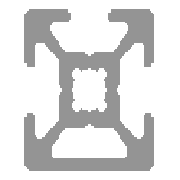
# Autodesk Inventor part: 3 842 992 889-2mm
Saved by Autodesk Inventor 2011 SP1 (Build 150282100, 282)
## iProperties
Created: 2011-02-10
Part Number: 3 842 992 889-2mm
Document SubType Name: Modeling
Designer: S. Wile
Density: 2.71 g/cm^3
Categories: <MemberInstance><Categories><Category DisplayName="Structural Shapes" InternalName="089c4875-fa83-4c05-b084-43b9cc11f5ed" Mnemonic="GRDR"><CategoryParameter DisplayName="Custom Base Point" InternalName="4f1d1b73-316d-484b-a3df-9cbabb16eb77" Mnemonic="shpBasePoint"/><CategoryParameter DisplayName="FG Authored" InternalName="9c666724-f362-4ea7-ac62-f6a007de5c69" Mnemonic="shpFGAuto"/><CategoryParameter DisplayName="Legacy Member ID" InternalName="340afe4f-75d7-48d3-ab7d-943f3c3da468" Mnemonic="LegacyMemberID"/><CategoryParameter DisplayName="Base Length" InternalName="42e34263-8f20-4d0e-ad48-bf1385b87c24" Mnemonic="shplen"/><CategoryParameter DisplayName="Distance of the Center of Gravity X-X" InternalName="26c9bdb8-9c79-4b4f-a92e-8e197583c9c4" Mnemonic="grcendistX"/><CategoryParameter DisplayName="Distance of the Center of Gravity Y-Y" InternalName="bcc4fb17-7af4-436a-8f8c-d0aa3b0248c5" Mnemonic="grcendistY"/><CategoryParameter DisplayName="Torsional Rigidity Modulus" InternalName="26c1ec35-5026-4c63-ad0a-751cf684a536" Mnemonic="torrigmod"/><CategoryParameter DisplayName="Torsional Section Modulus" InternalName="7c55a8dc-8844-49f9-a867-cc677b30ec9a" Mnemonic="torsecmod"/><CategoryParameter DisplayName="Coefficient of Shear Displacement" InternalName="de4c90c6-aaa8-468f-a335-6737b311b5d3" Mnemonic="shdispc"/><CategoryParameter DisplayName="Section Area" InternalName="1ff91680-64b0-4202-b9a3-7fd3f94bba3b" Mnemonic="secarea"/><CategoryParameter DisplayName="Moment of Inertia (x)" InternalName="4cd780bc-73d7-43ac-917a-579e5cbd684d" Mnemonic="inermomx"/><CategoryParameter DisplayName="Moment of Inertia (y)" InternalName="4b9f58ea-bced-460e-81ea-3d29ca5a49e3" Mnemonic="inermomy"/><CategoryParameter DisplayName="Section Module (x)" InternalName="72cfad18-cf51-4ed4-aaa7-c6b224f8419f" Mnemonic="secmodx"/><CategoryParameter DisplayName="Section Module (y)" InternalName="59eaa5e9-d227-48dc-b6c1-6920f96e0f95" Mnemonic="secmody"/><CategoryParameter DisplayName="Radius of Gyration (x)" InternalName="25778675-03e9-40c1-b6a8-4a9ed693320d" Mnemonic="gyrradx"/><CategoryParameter DisplayName="Radius of Gyration (y)" InternalName="bfa18ebe-1636-4dbe-8d42-b263e0b73184" Mnemonic="gyrrady"/><CategoryParameter DisplayName="Shape Thickness" InternalName="d109cf76-8eb4-42fc-9800-4409734adc67" Mnemonic="shpthick"/><CategoryParameter DisplayName="Second Shape Thickness" InternalName="9251a8e1-85fd-4e47-af99-afdb762317d9" Mnemonic="shpthick2"/><CategoryParameter DisplayName="Shape Width" InternalName="7c717d54-a18f-4666-b4d4-573cce22c62c" Mnemonic="shpwdth"/><CategoryParameter DisplayName="Shape Height" InternalName="50274e7d-5ac0-4796-92cb-c59e54983c67" Mnemonic="shpheig"/><CategoryParameter DisplayName="Mass per Length Unit" InternalName="0bb95a10-148f-4027-a459-38d7b056702a" Mnemonic="shpmass"/><CategoryParameter DisplayName="Section Designation" InternalName="5a64d034-428d-49c8-ba32-7619764de20f" Mnemonic="shpdes"/><Category DisplayName="Other" InternalName="f02205ff-2390-476f-921c-0b3185f88e84" Mnemonic="OTHSHP"><CategoryParameter DisplayName="Moment of Inertia (x)" InternalName="ec6737bc-264f-43ed-b0bd-f6d410c2718d" Mnemonic="inermomx"/><CategoryParameter DisplayName="Moment of Inertia (y)" InternalName="044c654e-f649-48ac-84cc-650a29ae31ca" Mnemonic="inermomy"/><CategoryParameter DisplayName="Section Module (x)" InternalName="cac70804-9d39-43bb-be17-56ea1f39a6c2" Mnemonic="secmodx"/><CategoryParameter DisplayName="Section Module (y)" InternalName="88b8bff9-a616-4028-93d5-ed4f79680d13" Mnemonic="secmody"/><CategoryParameter DisplayName="Section Area" InternalName="c46ecdf8-b6eb-4db9-8b25-30258930c1e3" Mnemonic="secarea"/><CategoryParameter DisplayName="Radius of Gyration (x)" InternalName="ee72c61e-565e-4fd6-b448-66e1e1abcb7e" Mnemonic="gyrradx"/><CategoryParameter DisplayName="Radius of Gyration (y)" InternalName="743e1dfe-1bba-408b-b985-cf752b207386" Mnemonic="gyrrady"/><CategoryParameter DisplayName="Shape Thickness" InternalName="12b1a788-9233-48fd-a933-2df8ff42b15f" Mnemonic="shpthick"/><CategoryParameter DisplayName="Mass per Length Unit" InternalName="2fd289d6-9394-4d2d-97e6-6659d7d4551d" Mnemonic="shpmass"/></Category></Category></Categories><FamilyTemplate Id="20x20-3S"><FamilyTemplateParameters><FamilyTemplateParameter ObjectType="kUserParameterObject" ValueType="xs:double" Id="1" ObjectReferenceKey="G_L"/><FamilyTemplateParameter ObjectType="kUserParameterObject" ValueType="xs:double" Id="2" ObjectReferenceKey="G_OFFSET_END"/><FamilyTemplateParameter ObjectType="kUserParameterObject" ValueType="xs:double" Id="3" ObjectReferenceKey="G_OFFSET_START"/><FamilyTemplateParameter ObjectType="kUserParameterObject" ValueType="xs:double" Id="4" ObjectReferenceKey="Length"/><FamilyTemplateParameter ObjectType="kPropertyObject" ValueType="xs:string" Id="7" ObjectReferenceKey="{32853F0F-3444-11d1-9E93-0060B03C1CA6}" SubObjectId="52"/><FamilyTemplateParameter ObjectType="kPartComponentDefinitionObject" ValueType="xs:string" Id="8" SubObjectId="Material"/><FamilyTemplateParameter ObjectType="kPropertyObject" ValueType="xs:string" Id="9" ObjectReferenceKey="{32853F0F-3444-11d1-9E93-0060B03C1CA6}" SubObjectId="5"/><FamilyTemplateParameter ObjectType="kPropertyObject" ValueType="xs:string" Id="10" ObjectReferenceKey="{32853F0F-3444-11D1-9E93-0060B03C1CA6}" SubObjectId="55"/><FamilyTemplateParameter ObjectType="kiPartTableColumnObject" ValueType="xs:string" Id="21" ObjectReferenceKey="FILENAME"/><FamilyTemplateParameter ObjectType="kiPartTableColumnObject" ValueType="xs:string" Id="22" ObjectReferenceKey="MEMBER_REVISION"/></FamilyTemplateParameters></FamilyTemplate><CategoryParameterMap><ParamToTemplateMap><ParamToTemplate CategoryParameter="//CategoryParameter[@InternalName='9c666724-f362-4ea7-ac62-f6a007de5c69']" ConstantValue="1"/><ParamToTemplate CategoryParameter="//CategoryParameter[@InternalName='2675968c-4ce5-49e0-a4f5-552d29089031']" TemplateParameter="7"/><ParamToTemplate CategoryParameter="//CategoryParameter[@InternalName='8b46a4cc-9585-4fed-90c3-899f57e09a73']" TemplateParameter="21"/><ParamToTemplate CategoryParameter="//CategoryParameter[@InternalName='42e34263-8f20-4d0e-ad48-bf1385b87c24']" TemplateParameter="4"/><ParamToTemplate CategoryParameter="//CategoryParameter[@InternalName='818a152a-d3c3-49ca-80ee-df7d91421b8e']" TemplateParameter="8"/><ParamToTemplate CategoryParameter="//CategoryParameter[@InternalName='a65d44b9-392f-4f4f-857b-e4b3d54996fe']" TemplateParameter="22"/><ParamToTemplate CategoryParameter="//CategoryParameter[@InternalName='016b6077-bfbe-49bd-92c9-d8d59c39c941']" TemplateParameter="9"/></ParamToTemplateMap></CategoryParameterMap></MemberInstance>
Stock Number: 3 842 992 889
Description: PROFILE 20x20 3S, -/-
Material: Aluminum-6061
Mass: 0.942693 g
Surface Area: 7.19171 cm^2
Volume: 0.347857 cm^3
Author: S. Wile
Autodesk Inventor part; units mm, degrees
ref_plane "YZ Plane" through (0, 0, 0) normal (1, 0, 0) x (0, 1, 0)
ref_plane "XZ Plane" through (0, 0, 0) normal (0, 1, 0) x (-1, 0, 0)
ref_plane "XY Plane" through (0, 0, 0) normal (0, 0, 1) x (1, 0, 0)
sketch "20x20-3S" plane through (0, 0, 0) normal (0, 0, 1) x (1, 0, 0)
  arc A0 (45.4955, 77.845) -> (45.5955, 77.8718) centre (45.4955, 78.045) ccw
  line L0 (45.4955, 77.845) -> (43.2168, 77.845)
  arc A1 (43.2168, 77.845) -> (42.8633, 77.6986) centre (43.2168, 77.345) ccw
  line L1 (42.8633, 77.6986) -> (40.5955, 75.4308)
  arc A2 (40.5955, 75.4308) -> (40.4491, 75.0772) centre (40.9491, 75.0772) ccw
  line L2 (40.4491, 75.0772) -> (40.4491, 74.345)
  arc A3 (40.4491, 74.345) -> (40.9491, 73.845) centre (40.9491, 74.345) ccw
  line L3 (40.9491, 73.845) -> (51.9491, 73.845)
  arc A4 (51.9491, 73.845) -> (52.4491, 74.345) centre (51.9491, 74.345) ccw
  line L4 (52.4491, 74.345) -> (52.4491, 75.0772)
  line L5 (55.4491, 85.295) -> (55.7491, 85.295)
  arc A5 (54.9491, 85.795) -> (55.4491, 85.295) centre (55.4491, 85.795) ccw
  line L6 (54.9491, 87.845) -> (54.9491, 85.795)
  arc A6 (54.9491, 87.845) -> (54.4491, 88.345) centre (54.4491, 87.845) ccw
  line L7 (53.7168, 88.345) -> (54.4491, 88.345)
  arc A7 (53.7168, 88.345) -> (53.3633, 88.1986) centre (53.7168, 87.845) ccw
  line L8 (51.0955, 85.9308) -> (53.3633, 88.1986)
  arc A8 (51.0955, 85.9308) -> (50.9491, 85.5772) centre (51.4491, 85.5772) ccw
  line L9 (50.9491, 83.2986) -> (50.9491, 85.5772)
  arc A9 (50.9223, 83.1986) -> (50.9491, 83.2986) centre (50.7491, 83.2986) ccw
  line L10 (50.4872, 82.445) -> (50.9223, 83.1986)
  arc A10 (50.4872, 82.445) -> (50.4872, 82.245) centre (50.6604, 82.345) ccw
  line L11 (50.9223, 81.4914) -> (50.4872, 82.245)
  arc A11 (50.9491, 81.3914) -> (50.9223, 81.4914) centre (50.7491, 81.3914) ccw
  line L12 (50.9491, 79.1128) -> (50.9491, 81.3914)
  arc A12 (50.9491, 79.1128) -> (51.0955, 78.7592) centre (51.4491, 79.1128) ccw
  line L13 (53.3633, 76.4915) -> (51.0955, 78.7592)
  arc A13 (53.3633, 76.4915) -> (53.7168, 76.345) centre (53.7168, 76.845) ccw
  line L14 (54.4491, 76.345) -> (53.7168, 76.345)
  arc A14 (54.4491, 76.345) -> (54.9491, 76.845) centre (54.4491, 76.845) ccw
  line L15 (54.9491, 78.795) -> (54.9491, 76.845)
  arc A15 (55.4491, 79.295) -> (54.9491, 78.795) centre (55.4491, 78.795) ccw
  line L16 (55.7491, 79.295) -> (55.4491, 79.295)
  arc A16 (55.9491, 79.095) -> (55.7491, 79.295) centre (55.7491, 79.095) ccw
  line L17 (55.9491, 78.995) -> (55.9491, 79.095)
  arc A17 (55.9491, 78.995) -> (56.1491, 78.795) centre (56.1491, 78.995) ccw
  line L18 (56.2491, 78.795) -> (56.1491, 78.795)
  arc A18 (56.4491, 78.595) -> (56.2491, 78.795) centre (56.2491, 78.595) ccw
  line L19 (56.4491, 73.845) -> (56.4491, 78.595)
  arc A19 (54.9491, 72.345) -> (56.4491, 73.845) centre (54.9491, 73.845) ccw
  line L20 (37.9491, 72.345) -> (54.9491, 72.345)
  arc A20 (36.4491, 73.845) -> (37.9491, 72.345) centre (37.9491, 73.845) ccw
  line L21 (36.4491, 78.595) -> (36.4491, 73.845)
  arc A21 (36.6491, 78.795) -> (36.4491, 78.595) centre (36.6491, 78.595) ccw
  line L22 (36.7491, 78.795) -> (36.6491, 78.795)
  arc A22 (36.7491, 78.795) -> (36.9491, 78.995) centre (36.7491, 78.995) ccw
  line L23 (36.9491, 79.095) -> (36.9491, 78.995)
  arc A23 (37.1491, 79.295) -> (36.9491, 79.095) centre (37.1491, 79.095) ccw
  line L24 (37.4491, 79.295) -> (37.1491, 79.295)
  arc A24 (37.9491, 78.795) -> (37.4491, 79.295) centre (37.4491, 78.795) ccw
  line L25 (37.9491, 76.845) -> (37.9491, 78.795)
  arc A25 (37.9491, 76.845) -> (38.4491, 76.345) centre (38.4491, 76.845) ccw
  line L26 (39.1813, 76.345) -> (38.4491, 76.345)
  arc A26 (39.1813, 76.345) -> (39.5349, 76.4915) centre (39.1813, 76.845) ccw
  line L27 (41.8026, 78.7592) -> (39.5349, 76.4915)
  arc A27 (41.8026, 78.7592) -> (41.9491, 79.1128) centre (41.4491, 79.1128) ccw
  line L28 (41.9491, 81.3914) -> (41.9491, 79.1128)
  arc A28 (41.9759, 81.4914) -> (41.9491, 81.3914) centre (42.1491, 81.3914) ccw
  line L29 (42.4109, 82.245) -> (41.9759, 81.4914)
  arc A29 (42.4109, 82.245) -> (42.4109, 82.445) centre (42.2377, 82.345) ccw
  line L30 (41.9759, 83.1986) -> (42.4109, 82.445)
  arc A30 (41.9491, 83.2986) -> (41.9759, 83.1986) centre (42.1491, 83.2986) ccw
  line L31 (41.9491, 85.5772) -> (41.9491, 83.2986)
  arc A31 (41.9491, 85.5772) -> (41.8026, 85.9308) centre (41.4491, 85.5772) ccw
  line L32 (39.5349, 88.1986) -> (41.8026, 85.9308)
  arc A32 (39.5349, 88.1986) -> (39.1813, 88.345) centre (39.1813, 87.845) ccw
  line L33 (38.4491, 88.345) -> (39.1813, 88.345)
  arc A33 (38.4491, 88.345) -> (37.9491, 87.845) centre (38.4491, 87.845) ccw
  line L34 (37.9491, 85.795) -> (37.9491, 87.845)
  arc A34 (37.4491, 85.295) -> (37.9491, 85.795) centre (37.4491, 85.795) ccw
  line L35 (37.1491, 85.295) -> (37.4491, 85.295)
  arc A35 (36.9491, 85.495) -> (37.1491, 85.295) centre (37.1491, 85.495) ccw
  line L36 (36.9491, 85.695) -> (36.9491, 85.495)
  arc A36 (36.9491, 85.695) -> (36.7491, 85.895) centre (36.7491, 85.695) ccw
  line L37 (36.6491, 85.895) -> (36.7491, 85.895)
  arc A37 (36.4491, 86.095) -> (36.6491, 85.895) centre (36.6491, 86.095) ccw
  line L38 (36.4491, 90.845) -> (36.4491, 86.095)
  arc A38 (37.9491, 92.345) -> (36.4491, 90.845) centre (37.9491, 90.845) ccw
  line L39 (42.6991, 92.345) -> (37.9491, 92.345)
  arc A39 (42.8991, 92.145) -> (42.6991, 92.345) centre (42.6991, 92.145) ccw
  line L40 (42.8991, 92.045) -> (42.8991, 92.145)
  arc A40 (42.8991, 92.045) -> (43.0991, 91.845) centre (43.0991, 92.045) ccw
  line L41 (43.2491, 91.845) -> (43.0991, 91.845)
  arc A41 (43.4491, 91.645) -> (43.2491, 91.845) centre (43.2491, 91.645) ccw
  line L42 (43.4491, 91.345) -> (43.4491, 91.645)
  arc A42 (42.9491, 90.845) -> (43.4491, 91.345) centre (42.9491, 91.345) ccw
  line L43 (40.9491, 90.845) -> (42.9491, 90.845)
  arc A43 (40.9491, 90.845) -> (40.4491, 90.345) centre (40.9491, 90.345) ccw
  line L44 (40.4491, 89.6128) -> (40.4491, 90.345)
  arc A44 (40.4491, 89.6128) -> (40.5955, 89.2592) centre (40.9491, 89.6128) ccw
  line L45 (42.8633, 86.9915) -> (40.5955, 89.2592)
  arc A45 (42.8633, 86.9915) -> (43.2168, 86.845) centre (43.2168, 87.345) ccw
  line L46 (45.4955, 86.845) -> (43.2168, 86.845)
  arc A46 (45.5955, 86.8182) -> (45.4955, 86.845) centre (45.4955, 86.645) ccw
  line L47 (46.3491, 86.3831) -> (45.5955, 86.8182)
  arc A47 (46.3491, 86.3831) -> (46.5491, 86.3831) centre (46.4491, 86.5563) ccw
  arc A48 (52.4491, 75.0772) -> (52.3026, 75.4308) centre (51.9491, 75.0772) ccw
  line L48 (52.3026, 75.4308) -> (50.0349, 77.6986)
  arc A49 (50.0349, 77.6986) -> (49.6813, 77.845) centre (49.6813, 77.345) ccw
  line L49 (49.6813, 77.845) -> (47.4027, 77.845)
  arc A50 (47.3027, 77.8718) -> (47.4027, 77.845) centre (47.4027, 78.045) ccw
  line L50 (47.3027, 77.8718) -> (46.5491, 78.3069)
  arc A51 (46.5491, 78.3069) -> (46.3491, 78.3069) centre (46.4491, 78.1337) ccw
  line L51 (46.3491, 78.3069) -> (45.5955, 77.8718)
  arc A52 (44.562, 85.2927) -> (43.5014, 84.2321) centre (46.4491, 82.345) ccw
  line L52 (43.5014, 84.2321) -> (44.0482, 83.5803)
  arc A53 (44.0482, 83.5803) -> (44.0482, 81.1097) centre (46.4491, 82.345) ccw
  line L53 (44.0482, 81.1097) -> (43.5014, 80.458)
  arc A54 (43.5014, 80.458) -> (44.562, 79.3973) centre (46.4491, 82.345) ccw
  line L54 (44.562, 79.3973) -> (45.2138, 79.9442)
  arc A55 (45.2138, 79.9442) -> (47.6844, 79.9442) centre (46.4491, 82.345) ccw
  line L55 (47.6844, 79.9442) -> (48.3361, 79.3973)
  arc A56 (48.3361, 79.3973) -> (49.3968, 80.458) centre (46.4491, 82.345) ccw
  line L56 (49.3968, 80.458) -> (48.8499, 81.1097)
  arc A57 (48.8499, 81.1097) -> (48.8499, 83.5803) centre (46.4491, 82.345) ccw
  line L57 (48.8499, 83.5803) -> (49.3968, 84.2321)
  arc A58 (49.3968, 84.2321) -> (48.3361, 85.2927) centre (46.4491, 82.345) ccw
  line L58 (48.3361, 85.2927) -> (47.6844, 84.7458)
  arc A59 (47.6844, 84.7458) -> (45.2138, 84.7458) centre (46.4491, 82.345) ccw
  line L59 (45.2138, 84.7458) -> (44.562, 85.2927)
  line L60 (47.3027, 86.8182) -> (46.5491, 86.3831)
  arc A60 (47.4027, 86.845) -> (47.3027, 86.8182) centre (47.4027, 86.645) ccw
  line L61 (49.6813, 86.845) -> (47.4027, 86.845)
  arc A61 (49.6813, 86.845) -> (50.0349, 86.9915) centre (49.6813, 87.345) ccw
  line L62 (52.3026, 89.2592) -> (50.0349, 86.9915)
  arc A62 (52.3026, 89.2592) -> (52.4491, 89.6128) centre (51.9491, 89.6128) ccw
  line L63 (52.4491, 90.345) -> (52.4491, 89.6128)
  arc A63 (52.4491, 90.345) -> (51.9491, 90.845) centre (51.9491, 90.345) ccw
  line L64 (49.9491, 90.845) -> (51.9491, 90.845)
  arc A64 (49.4491, 91.345) -> (49.9491, 90.845) centre (49.9491, 91.345) ccw
  line L65 (49.4491, 91.645) -> (49.4491, 91.345)
  arc A65 (49.6491, 91.845) -> (49.4491, 91.645) centre (49.6491, 91.645) ccw
  line L66 (49.7991, 91.845) -> (49.6491, 91.845)
  arc A66 (49.7991, 91.845) -> (49.9991, 92.045) centre (49.7991, 92.045) ccw
  line L67 (49.9991, 92.145) -> (49.9991, 92.045)
  arc A67 (50.1991, 92.345) -> (49.9991, 92.145) centre (50.1991, 92.145) ccw
  line L68 (54.9491, 92.345) -> (50.1991, 92.345)
  arc A68 (56.4491, 90.845) -> (54.9491, 92.345) centre (54.9491, 90.845) ccw
  line L69 (56.4491, 86.095) -> (56.4491, 90.845)
  arc A69 (56.2491, 85.895) -> (56.4491, 86.095) centre (56.2491, 86.095) ccw
  line L70 (56.1491, 85.895) -> (56.2491, 85.895)
  arc A70 (56.1491, 85.895) -> (55.9491, 85.695) centre (56.1491, 85.695) ccw
  line L71 (55.9491, 85.495) -> (55.9491, 85.695)
  arc A71 (55.7491, 85.295) -> (55.9491, 85.495) centre (55.7491, 85.495) ccw
sketch "Sketch1" plane through (0, 0, 0) normal (0, 0, 1) x (1, 0, 0)
  arc A0 (-0.9536, -4.5) -> (-0.8536, -4.4732) centre (-0.9536, -4.3) ccw
  line L0 (-0.9536, -4.5) -> (-3.2322, -4.5)
  arc A1 (-3.2322, -4.5) -> (-3.5858, -4.6464) centre (-3.2322, -5) ccw
  line L1 (-3.5858, -4.6464) -> (-5.8536, -6.9142)
  arc A2 (-5.8536, -6.9142) -> (-6, -7.2678) centre (-5.5, -7.2678) ccw
  line L2 (-6, -7.2678) -> (-6, -8)
  arc A3 (-6, -8) -> (-5.5, -8.5) centre (-5.5, -8) ccw
  line L3 (-5.5, -8.5) -> (5.5, -8.5)
  arc A4 (5.5, -8.5) -> (6, -8) centre (5.5, -8) ccw
  line L4 (6, -8) -> (6, -7.2678)
  line L5 (9, 2.95) -> (9.3, 2.95)
  arc A5 (8.5, 3.45) -> (9, 2.95) centre (9, 3.45) ccw
  line L6 (8.5, 5.5) -> (8.5, 3.45)
  arc A6 (8.5, 5.5) -> (8, 6) centre (8, 5.5) ccw
  line L7 (7.2678, 6) -> (8, 6)
  arc A7 (7.2678, 6) -> (6.9142, 5.8536) centre (7.2678, 5.5) ccw
  line L8 (4.6464, 3.5858) -> (6.9142, 5.8536)
  arc A8 (4.6464, 3.5858) -> (4.5, 3.2322) centre (5, 3.2322) ccw
  line L9 (4.5, 0.9536) -> (4.5, 3.2322)
  arc A9 (4.4732, 0.8536) -> (4.5, 0.9536) centre (4.3, 0.9536) ccw
  line L10 (4.0381, 0.1) -> (4.4732, 0.8536)
  arc A10 (4.0381, 0.1) -> (4.0381, -0.1) centre (4.2113, 0) ccw
  line L11 (4.4732, -0.8536) -> (4.0381, -0.1)
  arc A11 (4.5, -0.9536) -> (4.4732, -0.8536) centre (4.3, -0.9536) ccw
  line L12 (4.5, -3.2322) -> (4.5, -0.9536)
  arc A12 (4.5, -3.2322) -> (4.6464, -3.5858) centre (5, -3.2322) ccw
  line L13 (6.9142, -5.8536) -> (4.6464, -3.5858)
  arc A13 (6.9142, -5.8536) -> (7.2678, -6) centre (7.2678, -5.5) ccw
  line L14 (8, -6) -> (7.2678, -6)
  arc A14 (8, -6) -> (8.5, -5.5) centre (8, -5.5) ccw
  line L15 (8.5, -3.55) -> (8.5, -5.5)
  arc A15 (9, -3.05) -> (8.5, -3.55) centre (9, -3.55) ccw
  line L16 (9.3, -3.05) -> (9, -3.05)
  arc A16 (9.5, -3.25) -> (9.3, -3.05) centre (9.3, -3.25) ccw
  line L17 (9.5, -3.35) -> (9.5, -3.25)
  arc A17 (9.5, -3.35) -> (9.7, -3.55) centre (9.7, -3.35) ccw
  line L18 (9.8, -3.55) -> (9.7, -3.55)
  arc A18 (10, -3.75) -> (9.8, -3.55) centre (9.8, -3.75) ccw
  line L19 (10, -8.5) -> (10, -3.75)
  arc A19 (8.5, -10) -> (10, -8.5) centre (8.5, -8.5) ccw
  line L20 (-8.5, -10) -> (8.5, -10)
  arc A20 (-10, -8.5) -> (-8.5, -10) centre (-8.5, -8.5) ccw
  line L21 (-10, -3.75) -> (-10, -8.5)
  arc A21 (-9.8, -3.55) -> (-10, -3.75) centre (-9.8, -3.75) ccw
  line L22 (-9.7, -3.55) -> (-9.8, -3.55)
  arc A22 (-9.7, -3.55) -> (-9.5, -3.35) centre (-9.7, -3.35) ccw
  line L23 (-9.5, -3.25) -> (-9.5, -3.35)
  arc A23 (-9.3, -3.05) -> (-9.5, -3.25) centre (-9.3, -3.25) ccw
  line L24 (-9, -3.05) -> (-9.3, -3.05)
  arc A24 (-8.5, -3.55) -> (-9, -3.05) centre (-9, -3.55) ccw
  line L25 (-8.5, -5.5) -> (-8.5, -3.55)
  arc A25 (-8.5, -5.5) -> (-8, -6) centre (-8, -5.5) ccw
  line L26 (-7.2678, -6) -> (-8, -6)
  arc A26 (-7.2678, -6) -> (-6.9142, -5.8536) centre (-7.2678, -5.5) ccw
  line L27 (-4.6464, -3.5858) -> (-6.9142, -5.8536)
  arc A27 (-4.6464, -3.5858) -> (-4.5, -3.2322) centre (-5, -3.2322) ccw
  line L28 (-4.5, -0.9536) -> (-4.5, -3.2322)
  arc A28 (-4.4732, -0.8536) -> (-4.5, -0.9536) centre (-4.3, -0.9536) ccw
  line L29 (-4.0381, -0.1) -> (-4.4732, -0.8536)
  arc A29 (-4.0381, -0.1) -> (-4.0381, 0.1) centre (-4.2113, 0) ccw
  line L30 (-4.4732, 0.8536) -> (-4.0381, 0.1)
  arc A30 (-4.5, 0.9536) -> (-4.4732, 0.8536) centre (-4.3, 0.9536) ccw
  line L31 (-4.5, 3.2322) -> (-4.5, 0.9536)
  arc A31 (-4.5, 3.2322) -> (-4.6464, 3.5858) centre (-5, 3.2322) ccw
  line L32 (-6.9142, 5.8536) -> (-4.6464, 3.5858)
  arc A32 (-6.9142, 5.8536) -> (-7.2678, 6) centre (-7.2678, 5.5) ccw
  line L33 (-8, 6) -> (-7.2678, 6)
  arc A33 (-8, 6) -> (-8.5, 5.5) centre (-8, 5.5) ccw
  line L34 (-8.5, 3.45) -> (-8.5, 5.5)
  arc A34 (-9, 2.95) -> (-8.5, 3.45) centre (-9, 3.45) ccw
  line L35 (-9.3, 2.95) -> (-9, 2.95)
  arc A35 (-9.5, 3.15) -> (-9.3, 2.95) centre (-9.3, 3.15) ccw
  line L36 (-9.5, 3.35) -> (-9.5, 3.15)
  arc A36 (-9.5, 3.35) -> (-9.7, 3.55) centre (-9.7, 3.35) ccw
  line L37 (-9.8, 3.55) -> (-9.7, 3.55)
  arc A37 (-10, 3.75) -> (-9.8, 3.55) centre (-9.8, 3.75) ccw
  line L38 (-10, 8.5) -> (-10, 3.75)
  arc A38 (-8.5, 10) -> (-10, 8.5) centre (-8.5, 8.5) ccw
  line L39 (-3.75, 10) -> (-8.5, 10)
  arc A39 (-3.55, 9.8) -> (-3.75, 10) centre (-3.75, 9.8) ccw
  line L40 (-3.55, 9.7) -> (-3.55, 9.8)
  arc A40 (-3.55, 9.7) -> (-3.35, 9.5) centre (-3.35, 9.7) ccw
  line L41 (-3.2, 9.5) -> (-3.35, 9.5)
  arc A41 (-3, 9.3) -> (-3.2, 9.5) centre (-3.2, 9.3) ccw
  line L42 (-3, 9) -> (-3, 9.3)
  arc A42 (-3.5, 8.5) -> (-3, 9) centre (-3.5, 9) ccw
  line L43 (-5.5, 8.5) -> (-3.5, 8.5)
  arc A43 (-5.5, 8.5) -> (-6, 8) centre (-5.5, 8) ccw
  line L44 (-6, 7.2678) -> (-6, 8)
  arc A44 (-6, 7.2678) -> (-5.8536, 6.9142) centre (-5.5, 7.2678) ccw
  line L45 (-3.5858, 4.6464) -> (-5.8536, 6.9142)
  arc A45 (-3.5858, 4.6464) -> (-3.2322, 4.5) centre (-3.2322, 5) ccw
  line L46 (-0.9536, 4.5) -> (-3.2322, 4.5)
  arc A46 (-0.8536, 4.4732) -> (-0.9536, 4.5) centre (-0.9536, 4.3) ccw
  line L47 (-0.1, 4.0381) -> (-0.8536, 4.4732)
  arc A47 (-0.1, 4.0381) -> (0.1, 4.0381) centre (0, 4.2113) ccw
  arc A48 (6, -7.2678) -> (5.8536, -6.9142) centre (5.5, -7.2678) ccw
  line L48 (5.8536, -6.9142) -> (3.5858, -4.6464)
  arc A49 (3.5858, -4.6464) -> (3.2322, -4.5) centre (3.2322, -5) ccw
  line L49 (3.2322, -4.5) -> (0.9536, -4.5)
  arc A50 (0.8536, -4.4732) -> (0.9536, -4.5) centre (0.9536, -4.3) ccw
  line L50 (0.8536, -4.4732) -> (0.1, -4.0381)
  arc A51 (0.1, -4.0381) -> (-0.1, -4.0381) centre (0, -4.2113) ccw
  line L51 (-0.1, -4.0381) -> (-0.8536, -4.4732)
  arc A52 (-1.8871, 2.9477) -> (-2.9477, 1.8871) centre (0, 0) ccw
  line L52 (-2.9477, 1.8871) -> (-2.4008, 1.2353)
  arc A53 (-2.4008, 1.2353) -> (-2.4008, -1.2353) centre (0, 0) ccw
  line L53 (-2.4008, -1.2353) -> (-2.9477, -1.8871)
  arc A54 (-2.9477, -1.8871) -> (-1.8871, -2.9477) centre (0, 0) ccw
  line L54 (-1.8871, -2.9477) -> (-1.2353, -2.4008)
  arc A55 (-1.2353, -2.4008) -> (1.2353, -2.4008) centre (0, 0) ccw
  line L55 (1.2353, -2.4008) -> (1.8871, -2.9477)
  arc A56 (1.8871, -2.9477) -> (2.9477, -1.8871) centre (0, 0) ccw
  line L56 (2.9477, -1.8871) -> (2.4008, -1.2353)
  arc A57 (2.4008, -1.2353) -> (2.4008, 1.2353) centre (0, 0) ccw
  line L57 (2.4008, 1.2353) -> (2.9477, 1.8871)
  arc A58 (2.9477, 1.8871) -> (1.8871, 2.9477) centre (0, 0) ccw
  line L58 (1.8871, 2.9477) -> (1.2353, 2.4008)
  arc A59 (1.2353, 2.4008) -> (-1.2353, 2.4008) centre (0, 0) ccw
  line L59 (-1.2353, 2.4008) -> (-1.8871, 2.9477)
  line L60 (0.8536, 4.4732) -> (0.1, 4.0381)
  arc A60 (0.9536, 4.5) -> (0.8536, 4.4732) centre (0.9536, 4.3) ccw
  line L61 (3.2322, 4.5) -> (0.9536, 4.5)
  arc A61 (3.2322, 4.5) -> (3.5858, 4.6464) centre (3.2322, 5) ccw
  line L62 (5.8536, 6.9142) -> (3.5858, 4.6464)
  arc A62 (5.8536, 6.9142) -> (6, 7.2678) centre (5.5, 7.2678) ccw
  line L63 (6, 8) -> (6, 7.2678)
  arc A63 (6, 8) -> (5.5, 8.5) centre (5.5, 8) ccw
  line L64 (3.5, 8.5) -> (5.5, 8.5)
  arc A64 (3, 9) -> (3.5, 8.5) centre (3.5, 9) ccw
  line L65 (3, 9.3) -> (3, 9)
  arc A65 (3.2, 9.5) -> (3, 9.3) centre (3.2, 9.3) ccw
  line L66 (3.35, 9.5) -> (3.2, 9.5)
  arc A66 (3.35, 9.5) -> (3.55, 9.7) centre (3.35, 9.7) ccw
  line L67 (3.55, 9.8) -> (3.55, 9.7)
  arc A67 (3.75, 10) -> (3.55, 9.8) centre (3.75, 9.8) ccw
  line L68 (8.5, 10) -> (3.75, 10)
  arc A68 (10, 8.5) -> (8.5, 10) centre (8.5, 8.5) ccw
  line L69 (10, 3.75) -> (10, 8.5)
  arc A69 (9.8, 3.55) -> (10, 3.75) centre (9.8, 3.75) ccw
  line L70 (9.7, 3.55) -> (9.8, 3.55)
  arc A70 (9.7, 3.55) -> (9.5, 3.35) centre (9.7, 3.35) ccw
  line L71 (9.5, 3.15) -> (9.5, 3.35)
  arc A71 (9.3, 2.95) -> (9.5, 3.15) centre (9.3, 3.15) ccw
  constraints: 1 other
extrude "Extrusion3" add sketch "Sketch1" along normal blind 10
body "Solid2"
